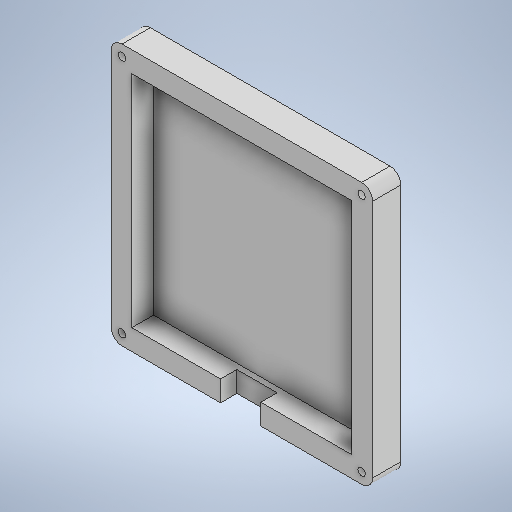
# Autodesk Inventor part: Bottom_Case_New
Saved by Autodesk Inventor 2025.1 (Build 291241000, 241)
## iProperties
Created: 2025-12-17
Part Number: Bottom_Case_New
Material: Generic
Document SubType Name: Modeling
Designer: omara
Density: 1 g/cm^3
Appearance: Default
Author: omara
Autodesk Inventor part; units mm, degrees
ref_plane "YZ Plane" through (0, 0, 0) normal (1, 0, 0) x (0, 1, 0)
ref_plane "XZ Plane" through (0, 0, 0) normal (0, 1, 0) x (-1, 0, 0)
sketch "Sketch1" plane through (0, 0, 0) normal (0, 0, 1) x (1, 0, 0)
  line L0 (0, 0) -> (101, 0)
  line L1 (101, 0) -> (101, 101)
  line L2 (101, 101) -> (0, 101)
  line L3 (0, 101) -> (0, 0)
  line L4 (-9.5, 110.5) -> (110.5, 110.5)
  line L5 (110.5, 110.5) -> (110.5, -9.5)
  line L6 (110.5, -9.5) -> (-9.5, -9.5)
  line L7 (-9.5, -9.5) -> (-9.5, 110.5)
  circle A0 centre (-4.5, 105.5) radius 1.7
  circle A1 centre (105.5, 105.5) radius 1.7
  circle A2 centre (105.5, -4.5) radius 1.7
  circle A3 centre (-4.5, -4.5) radius 1.7
  circle A4 centre (-4.5, -4.5) radius 3
  circle A5 centre (-4.5, 105.5) radius 3
  circle A6 centre (105.5, 105.5) radius 3
  circle A7 centre (105.5, -4.5) radius 3
  dimension "d0" = 101
  dimension "d1" = 101
  dimension "d2" = 120
  dimension "d3" = 120
  dimension "d4" = 9.5
  dimension "d5" = 9.5
  dimension "d6" = 3.4
  dimension "d7" = 3.4
  dimension "d8" = 3.4
  dimension "d9" = 3.4
  dimension "d10" = 5
  dimension "d11" = 5
  dimension "d12" = 5
  dimension "d13" = 5
  dimension "d14" = 5
  dimension "d15" = 5
  dimension "d16" = 5
  dimension "d17" = 5
  dimension "d18" = 6
  dimension "d19" = 6
  dimension "d20" = 6
  dimension "d21" = 6
  constraints: 16 end point, 8 centre point, 4 coincident, 4 parallel, 2 horizontal, 2 perpendicular
  measures "d0" distance of L2.end L1.end
  measures "d1" distance of L1.end L0.end
  measures "d2" distance of L5.end L6.end
  measures "d3" distance of L4.end L5.end
  measures "d4" distance between parallel lines of L4 L2
  measures "d5" distance between parallel lines of L7 L3
  measures "d6" diameter of A0
  measures "d7" diameter of A1
  measures "d8" diameter of A2
  measures "d9" diameter of A3
  measures "d10" distance from line of L7 A0.centre
  measures "d11" distance from line of L4 A0.centre
  measures "d12" distance from line of L5 A1.centre
  measures "d13" distance from line of L4 A1.centre
  measures "d14" distance from line of L5 A2.centre
  measures "d15" distance from line of L6 A2.centre
  measures "d16" distance from line of L6 A3.centre
  measures "d17" distance from line of L7 A3.centre
  measures "d18" diameter of A4
  measures "d19" diameter of A5
  measures "d20" diameter of A6
  measures "d21" diameter of A7
extrude "Extrusion1" add sketch "Sketch1" along normal blind 3 contours L3 L2 L1 L0
extrude "Extrusion2" add sketch "Sketch1" along normal blind 13 contours L4 L5 L6 L7
ref_plane "Work Plane2" through (0, 0, 3.1) normal (0, 0, -1) x (-1, 0, 0)
sketch "Sketch3" plane through (0, 0, 3) normal (0, 0, 1) x (1, 0, 0)
  circle A0 centre (-4.5, -4.5) radius 1.7 projected
  circle A1 centre (-4.5, -4.5) radius 3 projected
  circle A2 centre (105.5, -4.5) radius 1.7 projected
  circle A3 centre (105.5, -4.5) radius 3 projected
  circle A4 centre (105.5, 105.5) radius 3 projected
  circle A5 centre (105.5, 105.5) radius 1.7 projected
  circle A6 centre (-4.5, 105.5) radius 1.7 projected
  circle A7 centre (-4.5, 105.5) radius 3 projected
  point P0 (0, 0)
extrude "Extrusion4" add sketch "Sketch3" along normal blind 10
sketch "Sketch4" plane through (0, 0, 13) normal (0, 0, 1) x (1, 0, 0)
  line L0 (-9.5, -9.5) -> (110.5, -9.5) projected
  line L1 (101, 0) -> (0, 0) projected
  line L2 (59.245, -9.5) -> (40.745, -9.5)
  line L3 (40.745, -9.5) -> (40.745, 0)
  line L4 (40.745, 0) -> (59.245, 0)
  line L5 (59.245, 0) -> (59.245, -9.5)
  line L6 (110.5, -9.5) -> (110.5, 110.5) projected
  dimension "d32" = 18.5
  dimension "d33" = 51.255
  constraints: 8 end point, 2 parallel, 2 point on line, 1 horizontal, 1 perpendicular
  measures "d32" distance of L3.end L4.end
  measures "d33" distance between parallel lines of L6 L5
extrude "Extrusion5" cut sketch "Sketch4" against normal blind 7.5
fillet "Fillet1" radius 5 4 edges at (-9.5, 110.5, 6.5) (110.5, 110.5, 6.5) (110.5, -9.5, 6.5) (-9.5, -9.5, 6.5)
sketch "Sketch5" plane through (0, 0, 0) normal (0, 0, -1) x (-1, 0, 0)
  line L0 (-64.5, 108.5355) -> (-36.5, 108.5355) construction
  line L1 (-36.5, 108.5355) -> (-36.5, 104.5094) construction
  line L2 (-36.5, 104.5094) -> (-64.5, 104.5094) construction
  line L3 (-64.5, 104.5094) -> (-64.5, 108.5355) construction
  line L4 (-110.5, -4.5) -> (-110.5, 105.5) projected
  line L5 (9.5, 105.5) -> (9.5, -4.5) projected
  spline S0 degree 2 poles (-62.0349, 108.0514) (-61.862, 107.8488) (-61.6694, 107.256) (-61.6694, 106.8756) knots 0 0 0 1 2 2 2
  spline S1 degree 2 poles (-61.6694, 106.8756) (-61.6694, 106.5051) (-61.8571, 105.9049) (-62.0349, 105.7024) knots 0 0 0 1 2 2 2
  spline S2 degree 2 poles (-62.0349, 105.7024) (-62.2226, 105.49) (-62.7191, 105.2874) (-63.018, 105.2874) knots 0 0 0 1 2 2 2
  spline S3 degree 2 poles (-63.018, 105.2874) (-63.3267, 105.2874) (-63.8207, 105.4974) (-64.0011, 105.7024) knots 0 0 0 1 2 2 2
  spline S4 degree 2 poles (-64.0011, 105.7024) (-64.1764, 105.9049) (-64.3641, 106.5002) (-64.3641, 106.8756) knots 0 0 0 1 2 2 2
  spline S5 degree 2 poles (-64.3641, 106.8756) (-64.3641, 107.2585) (-64.174, 107.8414) (-63.9986, 108.0514) knots 0 0 0 1 2 2 2
  spline S6 degree 2 poles (-63.9986, 108.0514) (-63.8207, 108.2539) (-63.3243, 108.4639) (-63.018, 108.4639) knots 0 0 0 1 2 2 2
  spline S7 degree 2 poles (-63.018, 108.4639) (-62.7068, 108.4639) (-62.2078, 108.2465) (-62.0349, 108.0514) knots 0 0 0 1 2 2 2
  spline S8 degree 2 poles (-62.0917, 106.8756) (-62.0917, 107.177) (-62.2226, 107.6438) (-62.3412, 107.797) knots 0 0 0 1 2 2 2
  spline S9 degree 2 poles (-62.3412, 107.797) (-62.4622, 107.955) (-62.8031, 108.1131) (-63.0155, 108.1131) knots 0 0 0 1 2 2 2
  spline S10 degree 2 poles (-63.0155, 108.1131) (-63.2354, 108.1131) (-63.5663, 107.96) (-63.6923, 107.797) knots 0 0 0 1 2 2 2
  spline S11 degree 2 poles (-63.6923, 107.797) (-63.8133, 107.6414) (-63.9418, 107.172) (-63.9418, 106.8756) knots 0 0 0 1 2 2 2
  spline S12 degree 2 poles (-63.9418, 106.8756) (-63.9418, 106.2754) (-63.4379, 105.6382) (-63.0155, 105.6382) knots 0 0 0 1 2 2 2
  spline S13 degree 2 poles (-63.0155, 105.6382) (-62.5931, 105.6382) (-62.0917, 106.2754) (-62.0917, 106.8756) knots 0 0 0 1 2 2 2
  line L6 (-61.5533, 105.3516) -> (-60.5257, 108.3996)
  line L7 (-60.5257, 108.3996) -> (-60.0268, 108.3996)
  line L8 (-60.0268, 108.3996) -> (-58.9993, 105.3516)
  line L9 (-58.9993, 105.3516) -> (-59.4266, 105.3516)
  line L10 (-59.4266, 105.3516) -> (-59.7032, 106.2038)
  line L11 (-59.7032, 106.2038) -> (-60.8666, 106.2038)
  line L12 (-60.8666, 106.2038) -> (-61.1432, 105.3516)
  line L13 (-61.1432, 105.3516) -> (-61.5533, 105.3516)
  line L14 (-59.8144, 106.5496) -> (-60.2862, 107.9847)
  line L15 (-60.2862, 107.9847) -> (-60.7555, 106.5496)
  line L16 (-60.7555, 106.5496) -> (-59.8144, 106.5496)
  line L17 (-58.3497, 108.5355) -> (-58.4386, 107.3499)
  line L18 (-58.4386, 107.3499) -> (-58.7152, 107.3499)
  line L19 (-58.7152, 107.3499) -> (-58.8041, 108.5355)
  line L20 (-58.8041, 108.5355) -> (-58.3497, 108.5355)
  spline S14 degree 2 poles (-57.2382, 105.2973) (-57.4679, 105.2973) (-57.8655, 105.4208) (-57.9964, 105.49) knots 0 0 0 1 2 2 2
  line L21 (-57.9964, 105.49) -> (-57.9964, 105.9222)
  line L22 (-57.9964, 105.9222) -> (-57.9767, 105.9222)
  spline S15 degree 2 poles (-57.9767, 105.9222) (-57.9273, 105.8827) (-57.7939, 105.7888) (-57.6828, 105.737) knots 0 0 0 1 2 2 2
  spline S16 degree 2 poles (-57.6828, 105.737) (-57.5864, 105.69) (-57.3493, 105.6209) (-57.2233, 105.6209) knots 0 0 0 1 2 2 2
  spline S17 degree 2 poles (-57.2233, 105.6209) (-57.1319, 105.6209) (-56.922, 105.6629) (-56.8726, 105.6974) knots 0 0 0 1 2 2 2
  spline S18 degree 2 poles (-56.8726, 105.6974) (-56.801, 105.7444) (-56.7367, 105.8506) (-56.7367, 105.9593) knots 0 0 0 1 2 2 2
  spline S19 degree 2 poles (-56.7367, 105.9593) (-56.7367, 106.0951) (-56.8849, 106.2359) (-57.0751, 106.2828) knots 0 0 0 1 2 2 2
  spline S20 degree 2 poles (-57.0751, 106.2828) (-57.1492, 106.3001) (-57.3864, 106.3495) (-57.4876, 106.3767) knots 0 0 0 1 2 2 2
  spline S21 degree 2 poles (-57.4876, 106.3767) (-57.7494, 106.4533) (-57.9866, 106.7694) (-57.9866, 106.9942) knots 0 0 0 1 2 2 2
  spline S22 degree 2 poles (-57.9866, 106.9942) (-57.9866, 107.3054) (-57.5197, 107.6932) (-57.1344, 107.6932) knots 0 0 0 1 2 2 2
  spline S23 degree 2 poles (-57.1344, 107.6932) (-56.9442, 107.6932) (-56.5589, 107.5994) (-56.428, 107.5277) knots 0 0 0 1 2 2 2
  line L23 (-56.428, 107.5277) -> (-56.428, 107.1152)
  line L24 (-56.428, 107.1152) -> (-56.4477, 107.1152)
  spline S24 degree 2 poles (-56.4477, 107.1152) (-56.5959, 107.2338) (-56.9566, 107.3697) (-57.1418, 107.3697) knots 0 0 0 1 2 2 2
  spline S25 degree 2 poles (-57.1418, 107.3697) (-57.332, 107.3697) (-57.5938, 107.2091) (-57.5938, 107.0485) knots 0 0 0 1 2 2 2
  spline S26 degree 2 poles (-57.5938, 107.0485) (-57.5938, 106.9028) (-57.4382, 106.762) (-57.2653, 106.7176) knots 0 0 0 1 2 2 2
  spline S27 degree 2 poles (-57.2653, 106.7176) (-57.1813, 106.6953) (-56.9689, 106.6509) (-56.8528, 106.6237) knots 0 0 0 1 2 2 2
  spline S28 degree 2 poles (-56.8528, 106.6237) (-56.6009, 106.5595) (-56.344, 106.2656) (-56.344, 106.0111) knots 0 0 0 1 2 2 2
  spline S29 degree 2 poles (-56.344, 106.0111) (-56.344, 105.8629) (-56.4601, 105.6011) (-56.5737, 105.5048) knots 0 0 0 1 2 2 2
  spline S30 degree 2 poles (-56.5737, 105.5048) (-56.6947, 105.4035) (-57.0035, 105.2973) (-57.2382, 105.2973) knots 0 0 0 1 2 2 2
  line L25 (-52.0338, 105.3516) -> (-52.4389, 105.3516)
  line L26 (-52.4389, 105.3516) -> (-52.4389, 107.9773)
  line L27 (-52.4389, 107.9773) -> (-53.2343, 106.1915)
  line L28 (-53.2343, 106.1915) -> (-53.4813, 106.1915)
  line L29 (-53.4813, 106.1915) -> (-54.2692, 107.9773)
  line L30 (-54.2692, 107.9773) -> (-54.2692, 105.3516)
  line L31 (-54.2692, 105.3516) -> (-54.6471, 105.3516)
  line L32 (-54.6471, 105.3516) -> (-54.6471, 108.3996)
  line L33 (-54.6471, 108.3996) -> (-54.0938, 108.3996)
  line L34 (-54.0938, 108.3996) -> (-53.3331, 106.7027)
  line L35 (-53.3331, 106.7027) -> (-52.597, 108.3996)
  line L36 (-52.597, 108.3996) -> (-52.0338, 108.3996)
  line L37 (-52.0338, 108.3996) -> (-52.0338, 105.3516)
  spline S31 degree 2 poles (-50.1714, 105.5937) (-50.2184, 105.5591) (-50.3764, 105.4356) (-50.4505, 105.3986) knots 0 0 0 1 2 2 2
  spline S32 degree 2 poles (-50.4505, 105.3986) (-50.5518, 105.3442) (-50.742, 105.2874) (-50.9149, 105.2874) knots 0 0 0 1 2 2 2
  spline S33 degree 2 poles (-50.9149, 105.2874) (-51.0557, 105.2874) (-51.3101, 105.3936) (-51.4064, 105.49) knots 0 0 0 1 2 2 2
  spline S34 degree 2 poles (-51.4064, 105.49) (-51.4978, 105.5838) (-51.609, 105.8605) (-51.609, 106.0136) knots 0 0 0 1 2 2 2
  spline S35 degree 2 poles (-51.609, 106.0136) (-51.609, 106.2507) (-51.4089, 106.5867) (-51.1916, 106.683) knots 0 0 0 1 2 2 2
  spline S36 degree 2 poles (-51.1916, 106.683) (-50.9989, 106.7719) (-50.4752, 106.8386) (-50.1714, 106.8559) knots 0 0 0 1 2 2 2
  line L38 (-50.1714, 106.8559) -> (-50.1714, 106.93)
  spline S37 degree 2 poles (-50.1714, 106.93) (-50.1714, 107.0634) (-50.2529, 107.2289) (-50.327, 107.2758) knots 0 0 0 1 2 2 2
  spline S38 degree 2 poles (-50.327, 107.2758) (-50.4011, 107.3227) (-50.6136, 107.3524) (-50.7272, 107.3524) knots 0 0 0 1 2 2 2
  spline S39 degree 2 poles (-50.7272, 107.3524) (-50.8606, 107.3524) (-51.2212, 107.2733) (-51.4015, 107.1967) knots 0 0 0 1 2 2 2
  line L39 (-51.4015, 107.1967) -> (-51.4237, 107.1967)
  line L40 (-51.4237, 107.1967) -> (-51.4237, 107.5895)
  spline S40 degree 2 poles (-51.4237, 107.5895) (-51.3175, 107.6191) (-50.9199, 107.6932) (-50.7247, 107.6932) knots 0 0 0 1 2 2 2
  spline S41 degree 2 poles (-50.7247, 107.6932) (-50.4876, 107.6932) (-50.164, 107.6191) (-50.0356, 107.5228) knots 0 0 0 1 2 2 2
  spline S42 degree 2 poles (-50.0356, 107.5228) (-49.9096, 107.4289) (-49.7861, 107.1301) (-49.7861, 106.9152) knots 0 0 0 1 2 2 2
  line L41 (-49.7861, 106.9152) -> (-49.7861, 105.3516)
  line L42 (-49.7861, 105.3516) -> (-50.1714, 105.3516)
  line L43 (-50.1714, 105.3516) -> (-50.1714, 105.5937)
  line L44 (-50.1714, 105.9148) -> (-50.1714, 106.5496)
  spline S43 degree 2 poles (-50.1714, 106.5496) (-50.3098, 106.5373) (-50.7272, 106.4953) (-50.8581, 106.4557) knots 0 0 0 1 2 2 2
  spline S44 degree 2 poles (-50.8581, 106.4557) (-51.0112, 106.4088) (-51.2113, 106.2137) (-51.2113, 106.0408) knots 0 0 0 1 2 2 2
  spline S45 degree 2 poles (-51.2113, 106.0408) (-51.2113, 105.8432) (-50.989, 105.6431) (-50.7766, 105.6431) knots 0 0 0 1 2 2 2
  spline S46 degree 2 poles (-50.7766, 105.6431) (-50.5963, 105.6431) (-50.2999, 105.7987) (-50.1714, 105.9148) knots 0 0 0 1 2 2 2
  spline S47 degree 2 poles (-48.3362, 105.2998) (-48.5733, 105.2998) (-48.9661, 105.4455) (-49.1069, 105.5937) knots 0 0 0 1 2 2 2
  spline S48 degree 2 poles (-49.1069, 105.5937) (-49.2476, 105.7394) (-49.4033, 106.189) (-49.4033, 106.4903) knots 0 0 0 1 2 2 2
  spline S49 degree 2 poles (-49.4033, 106.4903) (-49.4033, 106.7917) (-49.2427, 107.2313) (-49.1069, 107.3795) knots 0 0 0 1 2 2 2
  spline S50 degree 2 poles (-49.1069, 107.3795) (-48.971, 107.5302) (-48.5684, 107.6908) (-48.3362, 107.6908) knots 0 0 0 1 2 2 2
  spline S51 degree 2 poles (-48.3362, 107.6908) (-48.1485, 107.6908) (-47.7978, 107.5845) (-47.6619, 107.5154) knots 0 0 0 1 2 2 2
  line L45 (-47.6619, 107.5154) -> (-47.6619, 107.0831)
  line L46 (-47.6619, 107.0831) -> (-47.6841, 107.0831)
  spline S52 degree 2 poles (-47.6841, 107.0831) (-47.7261, 107.1177) (-47.8546, 107.2066) (-47.946, 107.2536) knots 0 0 0 1 2 2 2
  spline S53 degree 2 poles (-47.946, 107.2536) (-48.0275, 107.2931) (-48.2448, 107.3548) (-48.3436, 107.3548) knots 0 0 0 1 2 2 2
  spline S54 degree 2 poles (-48.3436, 107.3548) (-48.6425, 107.3548) (-49.0056, 106.9028) (-49.0056, 106.4903) knots 0 0 0 1 2 2 2
  spline S55 degree 2 poles (-49.0056, 106.4903) (-49.0056, 106.0877) (-48.6548, 105.6357) (-48.3436, 105.6357) knots 0 0 0 1 2 2 2
  spline S56 degree 2 poles (-48.3436, 105.6357) (-48.1559, 105.6357) (-47.815, 105.7913) (-47.6841, 105.9123) knots 0 0 0 1 2 2 2
  line L47 (-47.6841, 105.9123) -> (-47.6619, 105.9123)
  line L48 (-47.6619, 105.9123) -> (-47.6619, 105.4801)
  spline S57 degree 2 poles (-47.6619, 105.4801) (-47.7187, 105.4529) (-47.8916, 105.3763) (-47.9608, 105.3591) knots 0 0 0 1 2 2 2
  spline S58 degree 2 poles (-47.9608, 105.3591) (-48.0596, 105.3294) (-48.2152, 105.2998) (-48.3362, 105.2998) knots 0 0 0 1 2 2 2
  line L49 (-46.0984, 107.2264) -> (-46.1181, 107.2264)
  spline S59 degree 2 poles (-46.1181, 107.2264) (-46.1626, 107.2387) (-46.2589, 107.2437) (-46.3256, 107.2437) knots 0 0 0 1 2 2 2
  spline S60 degree 2 poles (-46.3256, 107.2437) (-46.4812, 107.2437) (-46.7875, 107.1078) (-46.9258, 106.9744) knots 0 0 0 1 2 2 2
  line L50 (-46.9258, 106.9744) -> (-46.9258, 105.3516)
  line L51 (-46.9258, 105.3516) -> (-47.3112, 105.3516)
  line L52 (-47.3112, 105.3516) -> (-47.3112, 107.6389)
  line L53 (-47.3112, 107.6389) -> (-46.9258, 107.6389)
  line L54 (-46.9258, 107.6389) -> (-46.9258, 107.298)
  spline S61 degree 2 poles (-46.9258, 107.298) (-46.7159, 107.4857) (-46.4022, 107.6389) (-46.254, 107.6389) knots 0 0 0 1 2 2 2
  spline S62 degree 2 poles (-46.254, 107.6389) (-46.1947, 107.6389) (-46.1354, 107.6339) (-46.0984, 107.6265) knots 0 0 0 1 2 2 2
  line L55 (-46.0984, 107.6265) -> (-46.0984, 107.2264)
  spline S63 degree 2 poles (-43.9198, 106.4953) (-43.9198, 105.9173) (-44.4756, 105.2874) (-44.9399, 105.2874) knots 0 0 0 1 2 2 2
  spline S64 degree 2 poles (-44.9399, 105.2874) (-45.4167, 105.2874) (-45.9625, 105.937) (-45.9625, 106.4953) knots 0 0 0 1 2 2 2
  spline S65 degree 2 poles (-45.9625, 106.4953) (-45.9625, 107.0683) (-45.3994, 107.7031) (-44.9399, 107.7031) knots 0 0 0 1 2 2 2
  spline S66 degree 2 poles (-44.9399, 107.7031) (-44.4756, 107.7031) (-43.9198, 107.0708) (-43.9198, 106.4953) knots 0 0 0 1 2 2 2
  spline S67 degree 2 poles (-44.3175, 106.4953) (-44.3175, 106.9399) (-44.6411, 107.3721) (-44.9399, 107.3721) knots 0 0 0 1 2 2 2
  spline S68 degree 2 poles (-44.9399, 107.3721) (-45.2388, 107.3721) (-45.5649, 106.9399) (-45.5649, 106.4953) knots 0 0 0 1 2 2 2
  spline S69 degree 2 poles (-45.5649, 106.4953) (-45.5649, 106.063) (-45.2388, 105.6184) (-44.9399, 105.6184) knots 0 0 0 1 2 2 2
  spline S70 degree 2 poles (-44.9399, 105.6184) (-44.6435, 105.6184) (-44.3175, 106.0556) (-44.3175, 106.4953) knots 0 0 0 1 2 2 2
  spline S71 degree 2 poles (-41.6079, 106.557) (-41.6079, 105.984) (-42.1538, 105.3072) (-42.5712, 105.3072) knots 0 0 0 1 2 2 2
  spline S72 degree 2 poles (-42.5712, 105.3072) (-42.7416, 105.3072) (-43.0034, 105.3862) (-43.1393, 105.4677) knots 0 0 0 1 2 2 2
  line L56 (-43.1393, 105.4677) -> (-43.1393, 104.5094)
  line L57 (-43.1393, 104.5094) -> (-43.5246, 104.5094)
  line L58 (-43.5246, 104.5094) -> (-43.5246, 107.6389)
  line L59 (-43.5246, 107.6389) -> (-43.1393, 107.6389)
  line L60 (-43.1393, 107.6389) -> (-43.1393, 107.3993)
  spline S73 degree 2 poles (-43.1393, 107.3993) (-42.996, 107.5302) (-42.6453, 107.7031) (-42.4403, 107.7031) knots 0 0 0 1 2 2 2
  spline S74 degree 2 poles (-42.4403, 107.7031) (-42.0476, 107.7031) (-41.6079, 107.0807) (-41.6079, 106.557) knots 0 0 0 1 2 2 2
  spline S75 degree 2 poles (-42.0056, 106.5126) (-42.0056, 106.9053) (-42.255, 107.3375) (-42.5341, 107.3375) knots 0 0 0 1 2 2 2
  spline S76 degree 2 poles (-42.5341, 107.3375) (-42.6972, 107.3375) (-43.0034, 107.1918) (-43.1393, 107.0782) knots 0 0 0 1 2 2 2
  line L61 (-43.1393, 107.0782) -> (-43.1393, 105.779)
  spline S77 degree 2 poles (-43.1393, 105.779) (-42.9886, 105.7073) (-42.7737, 105.653) (-42.6354, 105.653) knots 0 0 0 1 2 2 2
  spline S78 degree 2 poles (-42.6354, 105.653) (-42.3365, 105.653) (-42.0056, 106.0927) (-42.0056, 106.5126) knots 0 0 0 1 2 2 2
  spline S79 degree 2 poles (-39.9332, 105.5937) (-39.9801, 105.5591) (-40.1382, 105.4356) (-40.2123, 105.3986) knots 0 0 0 1 2 2 2
  spline S80 degree 2 poles (-40.2123, 105.3986) (-40.3136, 105.3442) (-40.5038, 105.2874) (-40.6767, 105.2874) knots 0 0 0 1 2 2 2
  spline S81 degree 2 poles (-40.6767, 105.2874) (-40.8175, 105.2874) (-41.0719, 105.3936) (-41.1682, 105.49) knots 0 0 0 1 2 2 2
  spline S82 degree 2 poles (-41.1682, 105.49) (-41.2596, 105.5838) (-41.3708, 105.8605) (-41.3708, 106.0136) knots 0 0 0 1 2 2 2
  spline S83 degree 2 poles (-41.3708, 106.0136) (-41.3708, 106.2507) (-41.1707, 106.5867) (-40.9533, 106.683) knots 0 0 0 1 2 2 2
  spline S84 degree 2 poles (-40.9533, 106.683) (-40.7607, 106.7719) (-40.237, 106.8386) (-39.9332, 106.8559) knots 0 0 0 1 2 2 2
  line L62 (-39.9332, 106.8559) -> (-39.9332, 106.93)
  spline S85 degree 2 poles (-39.9332, 106.93) (-39.9332, 107.0634) (-40.0147, 107.2289) (-40.0888, 107.2758) knots 0 0 0 1 2 2 2
  spline S86 degree 2 poles (-40.0888, 107.2758) (-40.1629, 107.3227) (-40.3754, 107.3524) (-40.489, 107.3524) knots 0 0 0 1 2 2 2
  spline S87 degree 2 poles (-40.489, 107.3524) (-40.6224, 107.3524) (-40.983, 107.2733) (-41.1633, 107.1967) knots 0 0 0 1 2 2 2
  line L63 (-41.1633, 107.1967) -> (-41.1855, 107.1967)
  line L64 (-41.1855, 107.1967) -> (-41.1855, 107.5895)
  spline S88 degree 2 poles (-41.1855, 107.5895) (-41.0793, 107.6191) (-40.6816, 107.6932) (-40.4865, 107.6932) knots 0 0 0 1 2 2 2
  spline S89 degree 2 poles (-40.4865, 107.6932) (-40.2494, 107.6932) (-39.9258, 107.6191) (-39.7974, 107.5228) knots 0 0 0 1 2 2 2
  spline S90 degree 2 poles (-39.7974, 107.5228) (-39.6714, 107.4289) (-39.5479, 107.1301) (-39.5479, 106.9152) knots 0 0 0 1 2 2 2
  line L65 (-39.5479, 106.9152) -> (-39.5479, 105.3516)
  line L66 (-39.5479, 105.3516) -> (-39.9332, 105.3516)
  line L67 (-39.9332, 105.3516) -> (-39.9332, 105.5937)
  line L68 (-39.9332, 105.9148) -> (-39.9332, 106.5496)
  spline S91 degree 2 poles (-39.9332, 106.5496) (-40.0715, 106.5373) (-40.489, 106.4953) (-40.6199, 106.4557) knots 0 0 0 1 2 2 2
  spline S92 degree 2 poles (-40.6199, 106.4557) (-40.773, 106.4088) (-40.9731, 106.2137) (-40.9731, 106.0408) knots 0 0 0 1 2 2 2
  spline S93 degree 2 poles (-40.9731, 106.0408) (-40.9731, 105.8432) (-40.7508, 105.6431) (-40.5384, 105.6431) knots 0 0 0 1 2 2 2
  spline S94 degree 2 poles (-40.5384, 105.6431) (-40.3581, 105.6431) (-40.0617, 105.7987) (-39.9332, 105.9148) knots 0 0 0 1 2 2 2
  line L69 (-37.2483, 105.3516) -> (-37.6336, 105.3516)
  line L70 (-37.6336, 105.3516) -> (-37.6336, 105.5838)
  spline S95 degree 2 poles (-37.6336, 105.5838) (-37.7226, 105.5097) (-37.8535, 105.4109) (-37.9424, 105.3689) knots 0 0 0 1 2 2 2
  spline S96 degree 2 poles (-37.9424, 105.3689) (-38.0239, 105.3294) (-38.1993, 105.2874) (-38.3154, 105.2874) knots 0 0 0 1 2 2 2
  spline S97 degree 2 poles (-38.3154, 105.2874) (-38.5031, 105.2874) (-38.8192, 105.443) (-38.9304, 105.5937) knots 0 0 0 1 2 2 2
  spline S98 degree 2 poles (-38.9304, 105.5937) (-39.0415, 105.7444) (-39.165, 106.189) (-39.165, 106.478) knots 0 0 0 1 2 2 2
  spline S99 degree 2 poles (-39.165, 106.478) (-39.165, 106.7793) (-39.0094, 107.219) (-38.8736, 107.3845) knots 0 0 0 1 2 2 2
  spline S100 degree 2 poles (-38.8736, 107.3845) (-38.7476, 107.5327) (-38.3944, 107.7031) (-38.1993, 107.7031) knots 0 0 0 1 2 2 2
  spline S101 degree 2 poles (-38.1993, 107.7031) (-38.0288, 107.7031) (-37.7744, 107.6265) (-37.6336, 107.5475) knots 0 0 0 1 2 2 2
  line L71 (-37.6336, 107.5475) -> (-37.6336, 108.5355)
  line L72 (-37.6336, 108.5355) -> (-37.2483, 108.5355)
  line L73 (-37.2483, 108.5355) -> (-37.2483, 105.3516)
  line L74 (-37.6336, 105.9074) -> (-37.6336, 107.2289)
  spline S102 degree 2 poles (-37.6336, 107.2289) (-37.7769, 107.298) (-38.0041, 107.3499) (-38.135, 107.3499) knots 0 0 0 1 2 2 2
  spline S103 degree 2 poles (-38.135, 107.3499) (-38.4314, 107.3499) (-38.7674, 106.9053) (-38.7674, 106.4854) knots 0 0 0 1 2 2 2
  spline S104 degree 2 poles (-38.7674, 106.4854) (-38.7674, 106.0803) (-38.5105, 105.653) (-38.2264, 105.653) knots 0 0 0 1 2 2 2
  spline S105 degree 2 poles (-38.2264, 105.653) (-38.0758, 105.653) (-37.7695, 105.7913) (-37.6336, 105.9074) knots 0 0 0 1 2 2 2
  point P0 (0, 0)
  point P1 (-64.5, 106.5224)
  point P2 (-36.5, 106.5224)
  dimension "d37" = 46
  dimension "d38" = 46
  dimension "d39" = 4.0261
  dimension "d40" = 0.9906
  constraints: 2 midpoint, 1 parallel, 2 other
  measures "d37" distance from line of L4 point (-64.5, 106.522)
  measures "d38" distance from line of L5 point (-36.5, 106.522)
  measures "d39" distance between parallel lines of L2 L0
  measures "d40" distance from line of L5.start L2
extrude "Extrusion6" cut sketch "Sketch5" against normal blind 0.2
body "Solid1"
